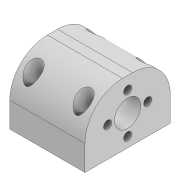
# Autodesk Inventor part: Nut holder
Saved by Autodesk Inventor 2020 (Build 240168000, 168)
## iProperties
Created: 2020-10-10
Part Number: Nut holder
Material: Generic
Document SubType Name: Modeling
Designer: ferrerx
Density: 1 g/cm^3
Appearance: Default
Author: ferrerx
Autodesk Inventor part; units mm, degrees
ref_plane "YZ Plane" through (0, 0, 0) normal (1, 0, 0) x (0, 1, 0)
ref_plane "XZ Plane" through (0, 0, 0) normal (0, 1, 0) x (-1, 0, 0)
ref_plane "XY Plane" through (0, 0, 0) normal (0, 0, 1) x (1, 0, 0)
sketch "Sketch1" plane through (0, 0, 0) normal (0, 1, 0) x (-1, 0, 0)
  line L0 (0, 0) -> (30, 0)
  line L1 (30, 0) -> (30, -34)
  line L2 (30, -34) -> (0, -34)
  line L3 (0, -34) -> (0, 0)
  dimension "d0" = 30
  dimension "d1" = 34
  constraints: 8 end point, 2 parallel, 1 horizontal, 1 perpendicular
  measures "d0" distance of L1.end L2.end
  measures "d1" distance of L2.end L0.start
extrude "Extrusion1" add sketch "Sketch1" along normal blind 25
sketch "Sketch2" plane through (0, 0, 0) normal (1, 0, 0) x (0, 0, -1)
  line L0 (34, 0) -> (0, 0) projected
  line L1 (17, 0) -> (17, 25) construction
  line L2 (34, 25) -> (0, 25) projected
  circle A0 centre (17, 12) radius 5.25
  circle A1 centre (17, 12) radius 10.2956 construction
  dimension "d4" = 10.5
  dimension "d5" = 12
  constraints: 2 centre point, 2 end point, 2 midpoint, 1 coincident, 1 point on line
  measures "d4" diameter of A0
  measures "d5" distance from line of L0 A0.centre
extrude "Extrusion2" cut sketch "Sketch2" against normal blind 30
sketch "Sketch3" plane through (0, 0, 0) normal (1, 0, 0) x (0, 0, -1)
  circle A0 centre (17, 12) radius 5.25 projected
  circle A1 centre (17, 12) radius 8 construction
  circle A2 centre (17, 20) radius 1.6
  point P0 (0, 0)
  dimension "d8" = 16
  dimension "d9" = 3.2
  constraints: 1 centre point, 1 coincident, 1 vertical alignment, 2 other
  measures "d9" diameter of A2
extrude "Extrusion3" cut sketch "Sketch3" against normal blind 30 contours A2
pattern_circular "Circular Pattern1" count 4 over 360 about axis through (0, 12, -17) along (-1, 0, 0) of "Extrusion3"
sketch "Sketch4" plane through (0, 25, 0) normal (0, 1, 0) x (1, 0, 0)
  line L0 (0, 0) -> (0, 34) projected
  line L1 (0, 17) -> (-30, 17) construction
  line L2 (-30, 34) -> (-30, 0) projected
  line L3 (-5, 4.5) -> (-25, 4.5) construction
  line L4 (-25, 4.5) -> (-25, 29.5) construction
  line L5 (-25, 29.5) -> (-5, 29.5) construction
  line L6 (-5, 29.5) -> (-5, 4.5) construction
  line L7 (-5, 4.5) -> (-25, 29.5) construction
  line L8 (-25, 4.5) -> (-5, 29.5) construction
  circle A0 centre (-25, 4.5) radius 1.55
  circle A1 centre (-25, 29.5) radius 1.55
  circle A2 centre (-5, 29.5) radius 1.55
  circle A3 centre (-5, 4.5) radius 1.55
  point P0 (-15, 17)
  dimension "d15" = 20
  dimension "d16" = 25
  dimension "d17" = 3.1
  dimension "d18" = 3.1
  dimension "d19" = 3.1
  dimension "d20" = 3.1
  constraints: 14 end point, 5 midpoint, 4 centre point, 4 coincident, 2 horizontal, 2 parallel, 1 perpendicular
  measures "d15" distance of L4.end L5.end
  measures "d16" distance of L5.end L3.start
  measures "d17" diameter of A0
  measures "d18" diameter of A1
  measures "d19" diameter of A2
  measures "d20" diameter of A3
extrude "Extrusion4" cut sketch "Sketch4" against normal blind 30
fillet "Fillet2" radius 15 2 edges at (-15, 25, -34) (-15, 25, 0)
sketch "Sketch7" plane through (0, 25, 0) normal (0, 1, 0) x (1, 0, 0)
  circle A0 centre (-25, 4.5) radius 1.55 projected
  circle A1 centre (-25, 4.5) radius 3
  circle A2 centre (-25, 29.5) radius 1.55 projected
  circle A3 centre (-25, 29.5) radius 3
  circle A4 centre (-5, 29.5) radius 1.55 projected
  circle A5 centre (-5, 29.5) radius 3
  circle A6 centre (-5, 4.5) radius 1.55 projected
  circle A7 centre (-5, 4.5) radius 3
  point P0 (0, 0)
  dimension "d46" = 6
  dimension "d47" = 6
  dimension "d48" = 6
  dimension "d49" = 6
  constraints: 4 centre point, 4 coincident
  measures "d46" diameter of A1
  measures "d47" diameter of A3
  measures "d48" diameter of A5
  measures "d49" diameter of A7
extrude "Extrusion7" cut sketch "Sketch7" against normal blind 11 contours A0 | A1 | A2 | A3 | A4 | A5 | A6 | A7
body "Solid1"
